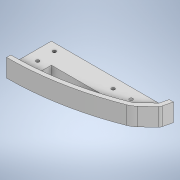
# Autodesk Inventor part: bumper_base_final _원본수정
Saved by Autodesk Inventor 2020 (Build 240168000, 168)
## iProperties
Created: 2022-06-30
Part Number: bumper_base_final _원본수정
Material: 일반
Document SubType Name: Modeling
Designer: samsung
Density: 1 g/cm^3
Appearance: 기본값
Author: samsung
Autodesk Inventor part; units mm, degrees
ref_plane "YZ Plane" through (0, 0, 0) normal (1, 0, 0) x (0, 1, 0)
ref_plane "XZ Plane" through (0, 0, 0) normal (0, 1, 0) x (-1, 0, 0)
ref_plane "XY Plane" through (0, 0, 0) normal (0, 0, 1) x (1, 0, 0)
sketch "스케치1" plane through (0, 0, 0) normal (0, 1, 0) x (-1, 0, 0)
  line L0 (-417.5, 136.0278) -> (167.5, 136.0278)
  line L1 (143.8982, 68.5278) -> (-85, 68.5278)
  line L2 (-165, 68.5278) -> (-381.3624, 68.5278)
  line L3 (-125, -531.4722) -> (-125, 1435.9267)
  circle A0 centre (-125, -531.4722) radius 1967.3989
  line L4 (-125, 111.6599) -> (186.953, 1411.0375)
  line L5 (-417.5444, 28.5399) -> (-411.5443, 53.4914)
  arc A1 (1441.9544, 38.2515) -> (-1691.7763, 38.7413) centre (-125, -531.4722) ccw
  line L6 (-371.3038, 78.1512) -> (-261.7019, 111.6599)
  line L7 (-261.7019, 111.6599) -> (11.7019, 111.6599)
  line L8 (-316.5029, 94.9056) -> (-320.1581, 106.8613)
  line L9 (-407.5098, 28.5399) -> (-405.1717, 38.2627)
  line L10 (-405.1717, 38.2627) -> (-402.8337, 47.9856)
  line L11 (-402.8337, 47.9856) -> (-371.3038, 78.1512)
  line L12 (-125, -531.4722) -> (-261.7019, 111.6599)
  line L13 (-125, -531.4722) -> (11.7019, 111.6599)
  line L14 (-417.5444, 28.5399) -> (-407.5098, 28.5399)
  line L15 (-125, -531.4722) -> (-371.3038, 78.1512)
  line L16 (-125, -531.4722) -> (121.3038, 78.1512)
  line L17 (11.7019, 111.6599) -> (121.3038, 78.1512)
  line L18 (167.4556, 28.5399) -> (156.6099, 73.7155)
  line L19 (157.5156, 28.5399) -> (148.4052, 66.4876)
  line L20 (121.3038, 78.1512) -> (152.8486, 47.9794)
  line L21 (155.1841, 38.2515) -> (1758.102, 38.2515)
  line L22 (155.1841, 38.2515) -> (164.5823, 40.5079)
  line L23 (157.5156, 28.5399) -> (167.4556, 28.5399)
  line L24 (155.1841, 38.2515) -> (1422.1711, 683.8137)
  line L25 (66.5029, 94.9056) -> (70.1581, 106.8613)
  line L26 (66.5029, 94.9056) -> (738.7616, 1236.1743)
  line L27 (66.5029, 94.9056) -> (147.3646, 1416.9826)
  line L28 (137.0762, 63.0653) -> (150.1137, 76.6961)
  line L29 (137.0762, 63.0653) -> (801.7772, 1203.965)
  line L30 (137.0762, 63.0653) -> (1307.7755, 816.7906)
  line L31 (-125, -531.4722) -> (148.4052, 66.4876)
  line L32 (-259.0118, 93.6599) -> (9.0118, 93.6599)
  line L33 (111.9521, 62.1879) -> (136.5817, 38.6304)
  line L34 (9.0118, 93.6599) -> (111.9521, 62.1879)
  line L35 (-361.9509, 62.1883) -> (-386.641, 38.5664)
  line L36 (-387.0049, 38.256) -> (-387.0101, 38.2515)
  line L37 (-388.9967, 28.5399) -> (-386.569, 38.6353)
  line L38 (-361.9509, 62.1883) -> (-259.0118, 93.6599)
  line L39 (-407.5098, 28.5399) -> (-388.9967, 28.5399)
  line L40 (136.5817, 38.6304) -> (139.0042, 28.5399)
  line L41 (157.5156, 28.5399) -> (139.0042, 28.5399)
  line L42 (-125, 111.6599) -> (-155, 111.6599)
  line L43 (-155, 93.6599) -> (-125, 93.6599)
  line L44 (-125, 93.6599) -> (-125, 111.6599)
  line L45 (-376.8352, 86.6988) -> (-411.5443, 53.4914)
  arc A2 (156.6099, 73.7155) -> (-376.8352, 86.6988) centre (-125, -531.4722) ccw
  arc A3 (148.4052, 66.4876) -> (-371.3038, 78.1512) centre (-125, -531.4722) ccw
  arc A4 (-398.3819, 66.4982) -> (-398.3844, 66.4971) centre (-125, -531.4722) ccw
  line L46 (-407.5098, 28.5399) -> (-402.8337, 47.9856)
  line L47 (-398.3829, 66.4939) -> (-398.3801, 66.5058)
  line L48 (-398.3844, 66.4971) -> (-398.2523, 66.2083)
  line L49 (-393.8505, 56.5801) -> (-125, -531.4722)
  line L50 (-125, 111.6599) -> (-135, 111.6599)
  line L51 (-135, 111.6599) -> (-135, 103.6599)
  line L52 (-135, 103.6599) -> (-125, 103.6599)
  line L53 (-316.5029, 94.9056) -> (-326.0659, 91.9818)
  line L54 (-326.0659, 91.9818) -> (-323.727, 84.3314)
  line L55 (-323.727, 84.3314) -> (-304.6009, 90.1788)
  line L56 (-304.6009, 90.1788) -> (-306.9398, 97.8293)
  line L57 (-402.8337, 47.9856) -> (-395.0554, 46.1151)
  line L58 (-395.0554, 46.1151) -> (-398.5625, 31.5309)
  line L59 (-398.5625, 31.5309) -> (-406.3408, 33.4013)
  line L60 (-387.0687, 63.0684) -> (-394.2944, 56.1554)
  line L61 (-394.2944, 56.1554) -> (-388.764, 50.3749)
  line L62 (-388.764, 50.3749) -> (-374.3127, 64.2009)
  line L63 (-374.3127, 64.2009) -> (-379.8431, 69.9814)
  line L64 (-165, 0) -> (-165, 124.81)
  line L65 (-341.215, 68.5278) -> (-341.215, 89.4604)
  line L66 (-388.9967, 28.5399) -> (-125, 28.5399)
  line L67 (-125, 0) -> (-165, 0)
  line L68 (-175, 28.5399) -> (-175, 124.1239)
  line L69 (-165, 0) -> (-135, 0)
  line L70 (-135, 0) -> (-135, 61.5)
  line L71 (-135, 61.5) -> (-165, 61.5)
  line L72 (-165, 61.5) -> (-165, 0)
  line L73 (-165, 61.5) -> (-175, 61.5)
  line L74 (-135, 61.5) -> (-125, 61.5)
  line L75 (-175, 78.5399) -> (-370.0325, 78.5399)
  line L76 (-165, 0) -> (-175, 0)
  line L77 (-175, 0) -> (-175, 28.5399)
  point P0 (0, 0)
  point P1 (0, 0)
  point P2 (143.8982, 61.5)
  point P3 (-393.8982, 61.5)
  point P4 (-417.5, 21.5)
  point P5 (-165, 0)
  point P6 (-85, 0)
  point P7 (-85, 12.4229)
  point P8 (167.5, 12.4229)
  point P9 (-393.8982, -388.5)
  point P10 (-165, -388.5)
  point P11 (167.5, -327)
  point P12 (-417.5, -327)
  point P13 (-85, -388.5)
  point P14 (143.8982, -388.5)
  point P15 (162, 21.5)
  point P16 (162, 12.4229)
  point P17 (167.5, 21.5)
  point P18 (-125, 0)
  point P19 (-125, 136.0278)
  point P20 (-125, 93.6599)
  point P21 (-125, 126.0278)
  point P22 (-317.2344, 97.2982)
  point P23 (-378.4524, 68.5278)
  point P24 (-393.0723, 54.878)
  point P25 (-175, 68.5278)
  point P26 (-341.215, 78.5399)
  point P27 (-125, 136.0278)
  point P28 (-385.9271, 39.2494)
  point P29 (-381.0308, 28.5399)
  dimension "d15" = 585
  dimension "d31" = 13.5
  dimension "d56" = 12
  dimension "d57" = 12
  dimension "d60" = 10
  dimension "d65" = 13.5
  dimension "d66" = 13.5
  dimension "d68" = 13.5
  dimension "d69" = 13.5
  dimension "d70" = 13.5
  dimension "d71" = 13.5
  dimension "d72" = 10
  dimension "d81" = 18
  dimension "d83" = 18
  dimension "d84" = 18
  dimension "d85" = 18
  dimension "d86" = 18
  dimension "d159" = 10
  dimension "d164" = 10
  dimension "d165" = 8
  dimension "d166" = 10
  dimension "d167" = 8
  dimension "d168" = 20
  dimension "d169" = 8
  dimension "d170" = 15
  dimension "d171" = 10
  dimension "d172" = 8
  dimension "d173" = 20
  dimension "d191" = 30
  dimension "d192" = 61.5
  dimension "d194" = 50
  constraints: 156 end point, 29 point on line, 21 perpendicular, 12 parallel, 11 horizontal, 9 point on circle, 7 midpoint, 3 centre point, 1 coincident, 1 tangent, 21 other
  measures "d15" distance of L18.start L5.start
  measures "d31" angle of L4 L3
  measures "d56" angle of L3 L12
  measures "d57" angle of L13 L3
  measures "d60" angle of L15 L12
  measures "d65" angle of L22 L21
  measures "d66" angle of L24 L22
  measures "d68" angle of L26 L25
  measures "d69" angle of L25 L27
  measures "d70" angle of L29 L28
  measures "d71" angle of L30 L28
  measures "d72" angle of L16 L13
  measures "d81" distance between parallel lines of L7 L32
  measures "d83" distance between parallel lines of L20 L33
  measures "d84" distance between parallel lines of L11 L35
  measures "d85" distance between parallel lines of L9 L37
  measures "d86" distance between parallel lines of L19 L40
  measures "d159" distance between parallel lines of L11 L45
  measures "d164" distance of L4.start L50.end
  measures "d165" distance of L50.end L51.end
  measures "d166" distance of L8.start L53.end
  measures "d167" distance of L53.end L54.end
  measures "d168" distance of L54.end L55.end
  measures "d169" distance of L10.end L57.end
  measures "d170" distance of L57.end L58.end
  measures "d171" distance of L60.start L60.end
  measures "d172" distance of L60.end L61.end
  measures "d173" distance of L61.end L62.end
  measures "d191" distance of L71.end L70.end
  measures "d192" distance of L70.end L69.end
  measures "d194" distance between parallel lines of L66 L75
extrude "돌출20" add sketch "스케치1" against normal blind 23 contours L3 A3 L8 A2 | L3 L7 L64 A3 | L8 A3 L11 L10 L9 L14 L5 L45 A2 | L3 L52 L51 L7 | L64 L7 L68 A3 | L3 L32 L64 L7 L51 L52 | L64 L32 L68 L7 | L65 L6 A3 | L3 L74 L71 L64 L32 | L64 L2 L68 L32 | L15 L2 L63 L11 | L6 L75 L65 L2 L15 | L65 L75 L6 | L3 L66 L70 L74 | L64 L73 L68 L2 | L75 L68 L2 L12 | L12 L2 L38 L75 | L63 L2 L11 | L15 L35 L49 L61 L62 L63 L2 | L2 L38 L35 L15 | L75 L38 L65 | L70 L66 L64 L71 | L68 L66 L12 L2 | L64 L66 L68 L73 | L12 L66 L15 L35 L38 L2 | L2 L63 L62 L61 L49 L11 | L15 L66 L49 L35 | L9 L59 L58 L57 L11 L61 L49 L35 L37 L39 | L66 L37 L35 L49 | L9 L10 L57 L58 L59 | L49 L61 L11
extrude "돌출21" add sketch "스케치1" along normal blind 20 contours L3 A3 L8 A2 | L8 A3 L11 L10 L9 L14 L5 L45 A2
sketch "스케치22" plane through (175, 0, 28.5399) normal (0, 0, -1) x (-1, 0, 0)
  line L0 (0, 0) -> (50, 0)
  line L1 (0, 0) -> (0, -23)
  line L2 (50, -23) -> (0, -23)
  line L3 (50, 0) -> (50, -23)
  line L4 (10, -10) -> (40, -10)
  line L5 (40, -10) -> (40, -23)
  line L6 (10, -23) -> (10, -10)
  point P0 (175, 0)
  point P1 (25, -23)
  dimension "d229" = 13
  dimension "d230" = 30
  constraints: 14 end point, 1 horizontal, 1 midpoint, 1 parallel, 1 perpendicular
  measures "d229" distance of L4.end L5.end
  measures "d230" distance of L4.start L4.end
extrude "돌출23" cut sketch "스케치22" against normal blind 32.96 contours L6 L4 L5 L2
sketch "스케치23" plane through (0, 0, 0) normal (0, 1, 0) x (1, 0, 0)
  line L0 (417.5444, -28.5399) -> (407.5098, -28.5399) projected
  line L1 (407.5098, -28.5399) -> (402.8337, -47.9856) projected
  line L2 (165, -28.5399) -> (135, -28.5399) projected
  line L3 (165, -28.5399) -> (165, -61.4999) projected
  line L4 (135, -28.5399) -> (135, -61.4999) projected
  line L5 (165, -61.4999) -> (135, -61.4999) projected
  point P0 (0, 0)
  point P1 (150, -46.4999)
  dimension "d257" = 15
  measures "d257" distance from line of L5 point (150, -46.5)
hole "구멍5" at (150, 0, 46.4999) direction (0, -1, 0) diameter 4.2 end through all counterbore diameter 8 counterbore depth 5
sketch "스케치24" plane through (0, 0, 0) normal (0, 1, 0) x (1, 0, 0)
  line L0 (417.5444, -28.5399) -> (407.5098, -28.5399) projected
  line L1 (175, -124.1239) -> (175, -78.5399) projected
  line L2 (341.215, -78.5399) -> (341.215, -89.4604) projected
  point P0 (0, 0)
  point P1 (150, -86.5)
  point P2 (341.215, -53.5399)
  point P3 (341.215, -84.0002)
  point P4 (298, -53.5399)
  dimension "d243" = 25
  dimension "d245" = 25
  dimension "d258" = 123
  constraints: 1 horizontal alignment, 1 midpoint, 1 vertical alignment
  measures "d243" distance from line of L1 point (150, -86.5)
  measures "d245" distance from line of point (341.215, -53.54) L0
  measures "d258" distance from line of point (298, -53.54) L1
hole "구멍6" at (150, 0, 86.5) at (341.215, 0, 53.5399) at (298, 0, 53.5399) direction (0, -1, 0) diameter 4.2 end through all counterbore diameter 8 counterbore depth 10
fillet "모깎기1" radius 50 1 edges at (376.8352, -1.5, 86.6988)
fillet "모깎기2" radius 10 1 edges at (411.5443, -1.5, 53.4914)
equation "\"d57\" = d56"
equation "\"d72\" = d60"
equation "\"d61\" = d60"
